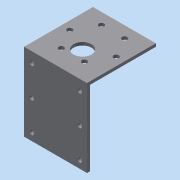
# Autodesk Inventor part: support_moteur
Saved by Autodesk Inventor 2016 (Build 200138000, 138)
## iProperties
Created: 2016-12-04
Part Number: support_moteur
Material: Generic
Document SubType Name: Modeling
Designer: Aegir
Density: 1 g/cm^3
Appearance: Default
Author: Aegir
Autodesk Inventor part; units mm, degrees
ref_plane "YZ Plane" through (0, 0, 0) normal (1, 0, 0) x (0, 1, 0)
ref_plane "XZ Plane" through (0, 0, 0) normal (0, 1, 0) x (-1, 0, 0)
ref_plane "XY Plane" through (0, 0, 0) normal (0, 0, 1) x (1, 0, 0)
sketch "Esquisse1" plane through (0, 0, 0) normal (0, 0, 1) x (1, 0, 0)
  circle A0 centre (0, 0) radius 18.4
  circle A1 centre (0, -7) radius 6
  circle A2 centre (15.5, 0) radius 1.25
  circle A3 centre (7.75, -13.4234) radius 1.25
  circle A4 centre (-7.75, -13.4234) radius 1.25
  circle A5 centre (-15.5, 0) radius 1.25
  circle A6 centre (-7.75, 13.4234) radius 1.25
  circle A7 centre (7.75, 13.4234) radius 1.25
  circle A8 centre (0, 15.5) radius 1.9
  circle A9 centre (-13.4234, -7.75) radius 1.9
  circle A10 centre (13.4234, -7.75) radius 1.9
  arc A11 (9.2253, -8.2857) -> (-9.2253, -8.2857) centre (0, 0) ccw
  spline S0 degree 3 poles (9.2254, -8.2857) (9.1718, -8.3454) (9.1113, -8.4012) (8.9929, -8.4831) (8.9346, -8.5143) (8.8333, -8.5456) (8.791, -8.5527) (8.7144, -8.5502) (8.6808, -8.5434) (8.6178, -8.5166) (8.59, -8.4975) (8.5381, -8.4462) (8.5162, -8.4136) (8.4741, -8.3274) (8.4589, -8.2705) (8.4364, -8.1241) (8.4381, -8.0284) (8.4482, -7.9376) knots 0 0 0 0 0.180455 0.180455 0.32493 0.32493 0.420837 0.420837 0.499135 0.499135 0.576434 0.576434 0.66484 0.66484 0.794052 0.794052 1 1 1 1
  arc A12 (8.4481, -7.9376) -> (-8.4481, -7.9376) centre (0, -7) ccw
  spline S1 degree 3 poles (-8.4482, -7.9376) (-8.4382, -8.0273) (-8.4365, -8.1217) (-8.4582, -8.2676) (-8.4733, -8.3251) (-8.5152, -8.412) (-8.537, -8.4449) (-8.5887, -8.4966) (-8.6164, -8.5158) (-8.6792, -8.543) (-8.7127, -8.5499) (-8.7891, -8.5529) (-8.8312, -8.546) (-8.932, -8.5155) (-8.99, -8.4848) (-9.1093, -8.403) (-9.1709, -8.3463) (-9.2254, -8.2857) knots 0 0 0 0 0.203505 0.203505 0.333659 0.333659 0.422431 0.422431 0.499705 0.499705 0.577923 0.577923 0.673342 0.673342 0.816724 0.816724 1 1 1 1
  line L0 (-21, 21) -> (21, 21)
  line L1 (21, 21) -> (21, -25)
  line L2 (21, -25) -> (-21, -25)
  line L3 (-21, -25) -> (-21, 21)
  circle A13 centre (-7.75, 13.4234) radius 1.75
  circle A14 centre (-15.5, 0) radius 1.75
  circle A15 centre (7.75, 13.4234) radius 1.75
  circle A16 centre (15.5, 0) radius 1.75
  circle A17 centre (-7.75, -13.4234) radius 1.75
  circle A18 centre (7.75, -13.4234) radius 1.75
  circle A19 centre (-7.75, 13.4234) radius 1.75
  circle A20 centre (7.75, 13.4234) radius 1.75
  circle A21 centre (15.5, 0) radius 1.75
  circle A22 centre (7.75, -13.4234) radius 1.75
  circle A23 centre (-7.75, -13.4234) radius 1.75
  circle A24 centre (-15.5, 0) radius 1.75
  circle A25 centre (0, -7) radius 6
extrude "Extrusion1" add sketch "Esquisse1" along normal blind 2 contours A0 | A8 | A9 | A10 | S0 A12 S1 A11 | L0 L1 L2 L3
sketch "Esquisse2" plane through (0, 0, 0) normal (0, 0, -1) x (-1, 0, 0)
  line L0 (-21, 21) -> (-21, -25) projected
  line L1 (21, -25) -> (-21, -25)
  line L2 (-21, -25) -> (-21, -23)
  line L3 (-21, -23) -> (21, -23)
  line L4 (21, -23) -> (21, -25)
  point P0 (0, 0)
  dimension "d7" = 2
  constraints: 8 end point, 2 parallel, 1 horizontal, 1 perpendicular, 1 point on line
  measures "d7" distance between parallel lines of L1 L3
extrude "Extrusion2" add sketch "Esquisse2" along normal blind 50
sketch "Esquisse3" plane through (-21, -25, 2) normal (0, -1, 0) x (1, 0, 0)
  line L0 (0, 0) -> (0, -52) projected
  line L1 (42, -52) -> (0, -52) projected
  point P0 (21, -2)
  point P1 (5, -47)
  point P2 (5, -27)
  point P3 (5, -7)
  point P4 (37, -47)
  point P5 (37, -27)
  point P6 (37, -7)
  dimension "d10" = 5
  dimension "d11" = 5
  dimension "d12" = 52
  dimension "d15" = 20
  dimension "d18" = 32
  constraints: 1 horizontal, 1 vertical, 5 other
  measures "d10" distance from line of L0 point (5, -47)
  measures "d11" distance from line of L1 point (5, -47)
  measures "d12" distance of L0.start L0.end
  measures "d15" distance of point (5, -47) point (5, -27)
  measures "d18" distance of point (5, -47) point (37, -47)
hole "Perçage1" at (-16, -25, -45) at (-16, -25, -25) at (-16, -25, -5) at (16, -25, -45) at (16, -25, -25) at (16, -25, -5) direction (0, 1, 0) diameter 3 end through all
